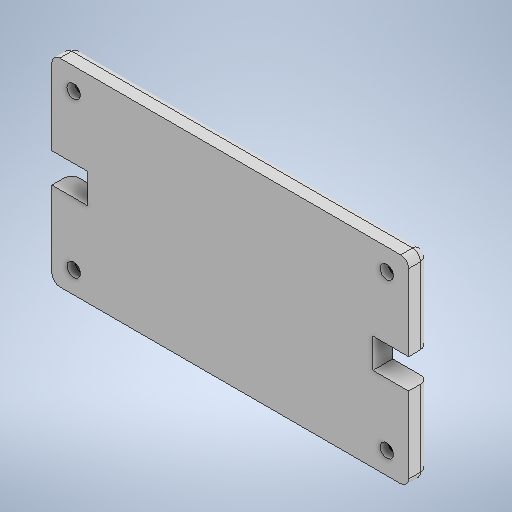
# Autodesk Inventor part: tcs3200_gate_lid
Saved by Autodesk Inventor 2025 (Build 290162000, 162)
## iProperties
Created: 2025-02-06
Part Number: tcs3200_gate_lid
Material: Všeobecné
Document SubType Name: Modeling
Designer: lukas
Density: 1 g/cm^3
Appearance: Výchozí
Author: lukas
## iProperties of the stored document tcs3200_gate_lid_3D tisk.ipt
Created: 2025-02-17
Part Number: tcs3200_gate_lid_3D tisk
Material: Všeobecné
Document SubType Name: Modeling
Designer: lukas
Density: 1 g/cm^3
Appearance: Výchozí
Author: lukas
Autodesk Inventor part; units mm, degrees
ref_plane "YZ Plane" through (0, 0, 0) normal (1, 0, 0) x (0, 1, 0)
ref_plane "XZ Plane" through (0, 0, 0) normal (0, 1, 0) x (-1, 0, 0)
ref_plane "XY Plane" through (0, 0, 0) normal (0, 0, 1) x (1, 0, 0)
sketch "Náčrt1" plane through (0, 0, 0) normal (0, 0, 1) x (1, 0, 0)
  line L0 (0, 35) -> (0, -35) projected
  line L1 (-63, 0) -> (63, 0) projected
  line L2 (-45, 25) -> (45, 25)
  line L3 (45, 25) -> (45, -25)
  line L4 (45, -25) -> (-45, -25)
  line L5 (-45, -25) -> (-45, 25)
  point P0 (0, 0)
  dimension "d0" = 90
  dimension "d1" = 50
  constraints: 8 end point, 2 parallel, 1 horizontal, 1 perpendicular, 2 other
  measures "d0" distance of L2.start L2.end
  measures "d1" distance of L2.end L3.end
extrude "Vysunutí1" add sketch "Náčrt1" along normal blind 5
sketch "Náčrt4" plane through (0, 0, 0) normal (0, 0, -1) x (-1, 0, 0)
  line L0 (45, 25) -> (45, -25) projected
  line L1 (-45, 25) -> (45, 25) projected
  line L2 (-45, -25) -> (-45, 25) projected
  line L3 (45, -25) -> (-45, -25) projected
  line L4 (0, -35) -> (0, 35) projected
  line L5 (-63, 0) -> (63, 0) projected
  point P0 (0, 0)
  point P1 (-39.5, 19.5)
  dimension "d13" = 5.5
  dimension "d14" = 5.5
  measures "d13" distance from line of L2 point (-39.5, 19.5)
  measures "d14" distance from line of L1 point (-39.5, 19.5)
hole "Díra1" at (39.5, 19.5, 0) direction (0, 0, 1) diameter 3.4 end through all counterbore diameter 6.1 counterbore depth 3 clearance for "Strojní šroub se zápustnou hlavou" size "M3" standard "Ansi M metrický profil"
mirror "Zrcadlit2" about plane through (0, 0, 0) normal (0, 1, 0) of "Díra1"
mirror "Zrcadlit3" about plane through (0, 0, 0) normal (1, 0, 0) of "Díra1", "Zrcadlit2"
fillet "Zaoblení2" radius 2 8 edges at (0, 25, 0) (45, 0, 0) (45, 25, 2.5) (0, -25, 0) (45, -25, 2.5) (-45, 0, 0) (-45, -25, 2.5) (-45, 25, 2.5)
sketch "Náčrt6" plane through (0, 0, 0) normal (0, 0, -1) x (-1, 0, 0)
  circle A0 centre (-39.5, 19.5) radius 3.05 projected
  circle A1 centre (-39.5, -19.5) radius 3.05 projected
  circle A2 centre (39.5, 19.5) radius 3.05 projected
  circle A3 centre (39.5, -19.5) radius 3.05 projected
  line L0 (43, -23) -> (-43, -23) projected
  line L1 (43, 23) -> (43, -23) projected
  line L2 (-43, 23) -> (43, 23) projected
  line L3 (-43, -23) -> (-43, 23) projected
  line L4 (-43, 23) -> (-45, 23) projected
  line L5 (-45, 23) -> (-45, -23) projected
  line L6 (-45, -23) -> (-43, -23) projected
  line L7 (-43, -23) -> (-43, 23) projected
  line L8 (-45, 3.75) -> (-36, 3.75)
  line L9 (-36, 3.75) -> (-36, -3.75)
  line L10 (-36, -3.75) -> (-45, -3.75)
  line L11 (-45, -3.75) -> (-45, 3.75)
  line L12 (-63, 0) -> (63, 0) projected
  point P0 (0, 0)
  dimension "d23" = 9
  dimension "d24" = 7.5
  constraints: 8 end point, 2 parallel, 1 horizontal, 1 perpendicular, 1 point on line, 1 other
  measures "d23" distance of L8.start L8.end
  measures "d24" distance between parallel lines of L8 L10
extrude "Vysunutí4" cut sketch "Náčrt6" against normal through all contours L10 L5 L12 L3 | L3 L12 L9 L10 | L12 L3 L8 L9 | L12 L5 L8 L3
mirror "Zrcadlit4" about plane through (0, 0, 0) normal (1, 0, 0) of "Vysunutí4"
sketch "Náčrt7" plane through (0, 0, 0) normal (0, 0, -1) x (-1, 0, 0)
  circle A0 centre (39.5, -19.5) radius 3.05 projected
  circle A1 centre (39.5, 19.5) radius 3.05 projected
  circle A2 centre (-39.5, -19.5) radius 3.05 projected
  circle A3 centre (-39.5, 19.5) radius 3.05 projected
  line L0 (43, -3.75) -> (36, -3.75) projected
  line L1 (36, -3.75) -> (36, 3.75) projected
  line L2 (36, 3.75) -> (43, 3.75) projected
  line L3 (43, 23) -> (43, 3.75) projected
  line L4 (-43, 23) -> (43, 23) projected
  line L5 (-43, 3.75) -> (-43, 23) projected
  line L6 (-43, 3.75) -> (-36, 3.75) projected
  line L7 (-36, 3.75) -> (-36, -3.75) projected
  line L8 (-36, -3.75) -> (-43, -3.75) projected
  line L9 (-43, -23) -> (-43, -3.75) projected
  line L10 (43, -23) -> (-43, -23) projected
  line L11 (43, -3.75) -> (43, -23) projected
  line L12 (43, 25) -> (-43, 25) projected
  line L13 (-43, -25) -> (43, -25) projected
  line L14 (-45, -3.75) -> (-45, -23) projected
  line L15 (45, -23) -> (45, -3.75) projected
  line L16 (45, 3.75) -> (45, 23) projected
  line L17 (-45, 23) -> (-45, 3.75) projected
  line L18 (0, -35) -> (0, 35) projected
  line L19 (-63, 0) -> (63, 0) projected
  line L20 (-12.75, 10) -> (12.75, 10)
  line L21 (12.75, 10) -> (12.75, -10)
  line L22 (12.75, -10) -> (-12.75, -10)
  line L23 (-12.75, -10) -> (-12.75, 10)
  line L24 (-10.75, 8) -> (10.75, 8)
  line L25 (10.75, 8) -> (10.75, -8)
  line L26 (10.75, -8) -> (-10.75, -8)
  line L27 (-10.75, -8) -> (-10.75, 8)
  line L28 (0, -8) -> (12.75, -8)
  line L29 (12.75, -8) -> (12.75, -10)
  line L30 (12.75, -10) -> (0, -10)
  line L31 (0, -10) -> (0, -8)
  line L32 (10.75, 0) -> (12.75, 0)
  line L33 (12.75, 0) -> (12.75, -10)
  line L34 (12.75, -10) -> (10.75, -10)
  line L35 (10.75, -10) -> (10.75, 0)
  point P0 (0, 0)
  dimension "d27" = 20
  dimension "d28" = 25.5
  dimension "d29" = 21.5
  dimension "d30" = 16
  constraints: 32 end point, 8 parallel, 4 horizontal, 4 perpendicular, 2 midpoint, 4 other
  measures "d27" distance between parallel lines of L22 L20
  measures "d28" distance of L20.start L20.end
  measures "d29" distance of L25.end L26.end
  measures "d30" distance of L24.end L25.end
extrude "Vysunutí5" add sketch "Náčrt7" along normal blind 8 contours L21 L28 L25 L19 | L19 L25 L24 L18 L20 L21 | L22 L23 L19 L27 L26 L18 | L18 L26 L35 L22 | L21 L22 L35 L28 | L18 L24 L27 L19 L23 L20
sketch "Náčrt8" plane through (12.75, -10, 0) normal (1, 0, 0) x (0, 0, -1)
  line L0 (0, 2) -> (0, 18) projected
  line L1 (0, 2) -> (8, 2) projected
  line L2 (8, 18) -> (8, 2) projected
  line L3 (0, 18) -> (8, 18) projected
  line L4 (8, 18) -> (0, 18)
  line L5 (0, 18) -> (0, 2)
  line L6 (0, 2) -> (8, 2)
  line L7 (8, 2) -> (8, 18)
  point P0 (0, 10)
  constraints: 8 end point, 2 parallel, 1 horizontal, 1 perpendicular
extrude "Vysunutí6" cut sketch "Náčrt8" against normal up to surface (2 mm away)
sketch "Náčrt9" plane through (12.75, 8, 0) normal (1, 0, 0) x (0, 0, -1)
  line L0 (8, -16) -> (0, -16) projected
  line L1 (0, -18) -> (0, -16) projected
  line L2 (0, -18) -> (8, -18) projected
  line L3 (8, -16) -> (8, -18) projected
  line L4 (0, 0) -> (8, 0) projected
  line L5 (8, 2) -> (8, 0) projected
  line L6 (0, 2) -> (8, 2) projected
  line L7 (0, 0) -> (0, 2) projected
  line L8 (4.5, 0) -> (6.5, 0)
  line L9 (6.5, 0) -> (6.5, 1)
  line L10 (6.5, 1) -> (4.5, 1)
  line L11 (4.5, 1) -> (4.5, 0)
  line L12 (-7.6, -8) -> (10.6, -8) projected
  point P0 (0, -8)
  dimension "d35" = 1
  dimension "d36" = 2
  dimension "d37" = 1.5
  constraints: 8 end point, 2 parallel, 1 horizontal, 1 perpendicular, 1 point on line
  measures "d35" distance of L8.end L9.end
  measures "d36" distance between parallel lines of L9 L11
  measures "d37" distance between parallel lines of L5 L9
extrude "Vysunutí7" cut sketch "Náčrt9" against normal up to surface (23.5 mm away) contours L11 L10 L9 L4
mirror "Zrcadlit5" about plane through (0, 0, 0) normal (0, 1, 0) of "Vysunutí7"
fillet "Zaoblení3" radius 2 2 edges at (-12.75, 10, -4) (-12.75, -10, -4)
